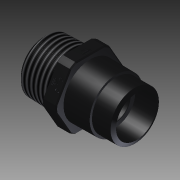
# Autodesk Inventor part: HSK-K 1.209.1201.70-Gland
Saved by Autodesk Inventor 2011 SP1 (Build 150282100, 282)
## iProperties
Created: 2018-02-18
Part Number: HSK-K 1.209.1201.70-Gland
Catalog Web Link: www.cadenas.de
Description: HSK-K NPT-Gland-Industrial cable glands
Vendor: SEALCON
Document SubType Name: Modeling
Designer: psAdmin
Manufacturer: SEALCON
Mass: 7.12094 g
Surface Area: 44.4321 cm^2
Volume: 7.12094 cm^3
Density: 1 g/cm^3
Category: PARTsolutions
Company: SEALCON
Title: HSK-K 1.209.1201.70-Gland
Author: Cadenas PARTsolutions
Comments: Industrial cable glands
PSOL_IDENT_0: {$CADENAS_DATA\23d-libs\sealcon\kabelverschraubungen\industriekabelverschraubungen\hsk_standard_kabe
PSOL_IDENT_1: lver\hsk_k\npt\hsk_k_npt_gland.prj},215 {VTYP=3D},{NB=HSK-K 1.209.1201.70-Gland},{LINA=HSK-K 1.209.1
PSOL_IDENT_2: 201.70-Gland},{NN=HSK-K NPT-Gland},{DATE=25.01.2018 07:57:44},{GEOMDATE=25.01.2018 07:44:49},{VERSIO
PSOL_IDENT_3: N=v121206082159},{LINEID=200},{LINESUBID=-1},{WBVAR=}  {NB=HSK-K 1.209.1201.70_gland},{LINA=HSK-K 1.
PSOL_IDENT_4: 209.1201.70_gland},{KT=DUMMY},{AG=1/2\" NPT},{FR=black},{GL=13},{H=27},{SW=24},{BN=1.209.1201.70},{C
PSOL_IDENT_5: OLX=0.04,0.04,0.04,0.00},{VER=2}
NN: HSK-K NPT-Gland
NT: Industrial cable glands
NB: HSK-K 1.209.1201.70-Gland
NBSYN: HSK-K $BN.-Gland
LINA: HSK-K 1.209.1201.70-Gland
AG: 1/2" NPT
FR: black
GL: 13
H: 27
SW: 24
BN: 1.209.1201.70
VER: 2
SUPPLIER: SEALCON
ARTICLENO: HSK-K 1.209.1201.70-Gland
BOMINFO: HSK-K 1.209.1201.70-Gland
CREATOR: CADENAS GmbH
Autodesk Inventor part; units mm, degrees
ref_plane "YZ Plane" through (0, 0, 0) normal (1, 0, 0) x (0, 1, 0)
ref_plane "XZ Plane" through (0, 0, 0) normal (0, 1, 0) x (-1, 0, 0)
ref_plane "XY Plane" through (0, 0, 0) normal (0, 0, 1) x (1, 0, 0)
sketch "Sketch_1" plane through (0, 0, 0) normal (0, 0, 1) x (1, 0, 0)
  line L0 (18, 0) -> (0, 0)
  line L1 (0, 0) -> (0, 8.75)
  line L2 (0, 8.75) -> (1.3401, 10.0901)
  line L3 (1.3401, 10.0901) -> (13, 10.4541)
  line L4 (13, 10.4541) -> (13, 13.2)
  line L5 (13, 13.2) -> (17.6, 13.2)
  line L6 (17.6, 13.2) -> (18, 12.8)
  line L7 (18, 12.8) -> (18, 0)
  line L8 (18, 0) -> (0, 0)
  constraints: 18 end point
revolve "Revolution1" add sketch "Sketch_1" angle 360 about axis through (18, 0, 0) along (1, 0, 0)
thread "Thread1" size "1/2" designation "1/2 - 14 NPT" standard "NPT" full length
sketch "Sketch_2" plane through (18, 0, 0) normal (1, 0, 0) x (0, 0, -1)
  line L0 (-24, -24) -> (24, -24)
  line L1 (24, -24) -> (24, 24)
  line L2 (24, 24) -> (-24, 24)
  line L3 (-24, 24) -> (-24, -24)
  line L4 (-12, -6.9282) -> (0, -13.8564)
  line L5 (0, -13.8564) -> (12, -6.9282)
  line L6 (12, -6.9282) -> (12, 6.9282)
  line L7 (12, 6.9282) -> (0, 13.8564)
  line L8 (0, 13.8564) -> (-12, 6.9282)
  line L9 (-12, 6.9282) -> (-12, -6.9282)
  constraints: 20 end point
extrude "Extrusion1" cut sketch "Sketch_2" against normal blind 5
sketch "Sketch_3" plane through (0, 0, 0) normal (0, 0, 1) x (1, 0, 0)
  line L0 (27.5, 0) -> (18, 0)
  line L1 (18, 0) -> (18, 10.325)
  line L2 (18, 10.325) -> (28, 10.225)
  line L3 (28, 10.225) -> (28, 9.35)
  line L4 (28, 9.35) -> (28.7, 9.35)
  line L5 (28.7, 9.35) -> (28.7, 7.85)
  line L6 (28.7, 7.85) -> (27.5, 7.85)
  line L7 (27.5, 7.85) -> (27.5, 0)
  line L8 (27.5, 0) -> (18, 0)
  constraints: 18 end point
revolve "Revolution2" add sketch "Sketch_3" angle 360 about axis through (27.5, 0, 0) along (1, 0, 0)
sketch "Sketch_5" plane through (0, 0, 0) normal (0, 0, 1) x (1, 0, 0)
  line L0 (28.5, 0) -> (-1, 0)
  line L1 (-1, 0) -> (-1, 7.4828)
  line L2 (-1, 7.4828) -> (0, 7.4828)
  arc A0 (0, 7.4828) -> (0.9826, 6.4829) centre (1, 7.4828) ccw
  line L3 (0.9826, 6.4829) -> (23, 6.1)
  line L4 (23, 6.1) -> (27.3, 6.1)
  arc A1 (27.3, 6.1) -> (27.5, 6.3) centre (27.3, 6.3) ccw
  line L5 (27.5, 6.3) -> (28.5, 6.3)
  line L6 (28.5, 6.3) -> (28.5, 0)
  line L7 (28.5, 0) -> (-1, 0)
  constraints: 16 end point, 4 point on circle, 2 centre point
revolve "Revolution3" cut sketch "Sketch_5" angle 360 about axis through (28.5, 0, 0) along (1, 0, 0)
sketch "Sketch_4" plane through (0, 0, 12) normal (0, 0, 1) x (1, 0, 0)
  line L0 (15.8137, 0.9977) -> (16.0537, 0.9977)
  line L1 (16.0537, 0.9977) -> (16.0537, -1.1725)
  arc A0 (16.0537, -1.1725) -> (17, -1.1725) centre (16.5269, -1.1725) ccw
  line L2 (17, -1.1725) -> (17, -1.0594)
  line L3 (17, -1.0594) -> (17.24, -1.0594)
  line L4 (17.24, -1.0594) -> (17.24, -0.936)
  line L5 (17.24, -0.936) -> (17, -0.936)
  line L6 (17, -0.936) -> (17, 1.1725)
  arc A1 (17, 1.1725) -> (16.0537, 1.1725) centre (16.5269, 1.1725) ccw
  line L7 (16.0537, 1.1725) -> (16.0537, 1.1211)
  line L8 (16.0537, 1.1211) -> (15.8137, 1.1211)
  line L9 (15.8137, 1.1211) -> (15.8137, 0.9977)
  arc A2 (16.1772, -1.1725) -> (16.8766, -1.1725) centre (16.5269, -1.1725) ccw
  line L10 (16.8766, -1.1725) -> (16.8766, -1.0594)
  line L11 (16.8766, -1.0594) -> (16.3596, -1.0594)
  line L12 (16.3596, -1.0594) -> (16.3596, -1.1211)
  line L13 (16.3596, -1.1211) -> (16.2937, -1.1211)
  line L14 (16.2937, -1.1211) -> (16.2937, -0.936)
  line L15 (16.2937, -0.936) -> (16.8766, -0.936)
  line L16 (16.8766, -0.936) -> (16.8766, 1.1725)
  arc A3 (16.8766, 1.1725) -> (16.1772, 1.1725) centre (16.5269, 1.1725) ccw
  line L17 (16.1772, 1.1725) -> (16.1772, 1.1211)
  line L18 (16.1772, 1.1211) -> (16.76, 1.1211)
  line L19 (16.76, 1.1211) -> (16.76, 0.9977)
  line L20 (16.76, 0.9977) -> (16.5598, 0.9977)
  line L21 (16.5598, 0.9977) -> (16.5598, 0.936)
  line L22 (16.5598, 0.936) -> (16.76, 0.936)
  line L23 (16.76, 0.936) -> (16.76, 0.8194)
  line L24 (16.76, 0.8194) -> (16.2937, 0.8194)
  line L25 (16.2937, 0.8194) -> (16.2937, 0.936)
  line L26 (16.2937, 0.936) -> (16.494, 0.936)
  line L27 (16.494, 0.936) -> (16.494, 0.9977)
  line L28 (16.494, 0.9977) -> (16.1772, 0.9977)
  line L29 (16.1772, 0.9977) -> (16.1772, -1.1725)
  constraints: 60 end point, 8 point on circle, 4 centre point
extrude "Extrusion2" cut sketch "Sketch_4" against normal blind 0.2
sketch "Sketch_8" plane through (0, 0, 12) normal (0, 0, 1) x (1, 0, 0)
  line L0 (16.2937, -0.8743) -> (16.3596, -0.8743)
  line L1 (16.3596, -0.8743) -> (16.3596, -0.8125)
  line L2 (16.3596, -0.8125) -> (16.494, -0.8125)
  line L3 (16.494, -0.8125) -> (16.494, -0.8743)
  line L4 (16.494, -0.8743) -> (16.5598, -0.8743)
  line L5 (16.5598, -0.8743) -> (16.5598, -0.8125)
  line L6 (16.5598, -0.8125) -> (16.6942, -0.8125)
  line L7 (16.6942, -0.8125) -> (16.6942, -0.8743)
  line L8 (16.6942, -0.8743) -> (16.76, -0.8743)
  line L9 (16.76, -0.8743) -> (16.76, -0.696)
  line L10 (16.76, -0.696) -> (16.2937, -0.696)
  line L11 (16.2937, -0.696) -> (16.2937, -0.8743)
  constraints: 24 end point
extrude "Extrusion3" cut sketch "Sketch_8" against normal blind 0.2
sketch "Sketch_9" plane through (0, 0, 12) normal (0, 0, 1) x (1, 0, 0)
  line L0 (16.2937, -0.264) -> (16.6942, -0.264)
  line L1 (16.6942, -0.264) -> (16.6942, -0.3257)
  line L2 (16.6942, -0.3257) -> (16.2937, -0.3257)
  line L3 (16.2937, -0.3257) -> (16.2937, -0.4491)
  line L4 (16.2937, -0.4491) -> (16.6942, -0.4491)
  line L5 (16.6942, -0.4491) -> (16.6942, -0.5108)
  line L6 (16.6942, -0.5108) -> (16.2937, -0.5108)
  line L7 (16.2937, -0.5108) -> (16.2937, -0.6343)
  line L8 (16.2937, -0.6343) -> (16.76, -0.6343)
  line L9 (16.76, -0.6343) -> (16.76, -0.1474)
  line L10 (16.76, -0.1474) -> (16.2937, -0.1474)
  line L11 (16.2937, -0.1474) -> (16.2937, -0.264)
  constraints: 24 end point
extrude "Extrusion4" cut sketch "Sketch_9" against normal blind 0.2
sketch "Sketch_10" plane through (0, 0, 12) normal (0, 0, 1) x (1, 0, 0)
  line L0 (16.2937, 0.0377) -> (16.2937, -0.0857)
  line L1 (16.2937, -0.0857) -> (16.76, -0.0857)
  line L2 (16.76, -0.0857) -> (16.76, 0.4011)
  line L3 (16.76, 0.4011) -> (16.2937, 0.4011)
  line L4 (16.2937, 0.4011) -> (16.2937, 0.2846)
  line L5 (16.2937, 0.2846) -> (16.6942, 0.2846)
  line L6 (16.6942, 0.2846) -> (16.6942, 0.2229)
  line L7 (16.6942, 0.2229) -> (16.2937, 0.2229)
  line L8 (16.2937, 0.2229) -> (16.2937, 0.0994)
  line L9 (16.2937, 0.0994) -> (16.6942, 0.0994)
  line L10 (16.6942, 0.0994) -> (16.6942, 0.0377)
  line L11 (16.6942, 0.0377) -> (16.2937, 0.0377)
  constraints: 24 end point
extrude "Extrusion5" cut sketch "Sketch_10" against normal blind 0.2
sketch "Sketch_11" plane through (0, 0, 12) normal (0, 0, 1) x (1, 0, 0)
  line L0 (16.2937, 0.7577) -> (16.2937, 0.4628)
  line L1 (16.2937, 0.4628) -> (16.76, 0.4628)
  line L2 (16.76, 0.4628) -> (16.76, 0.5794)
  line L3 (16.76, 0.5794) -> (16.3596, 0.5794)
  line L4 (16.3596, 0.5794) -> (16.3596, 0.6411)
  line L5 (16.3596, 0.6411) -> (16.76, 0.6411)
  line L6 (16.76, 0.6411) -> (16.76, 0.7577)
  line L7 (16.76, 0.7577) -> (16.2937, 0.7577)
  constraints: 16 end point
extrude "Extrusion6" cut sketch "Sketch_11" against normal blind 0.2
sketch "Sketch_12" plane through (0, -10.3923, 6) normal (0, 0.8660254, -0.5) x (1, 0, 0)
  arc A0 (16.2286, -1.6686) -> (16.2286, -2.0114) centre (16.2286, -1.84) ccw
  line L0 (16.2286, -2.0114) -> (16.7429, -2.0114)
  line L1 (16.7429, -2.0114) -> (16.7429, -1.9428)
  line L2 (16.7429, -1.9428) -> (16.2286, -1.9428)
  arc A1 (16.2286, -1.7371) -> (16.2286, -1.9428) centre (16.2286, -1.84) ccw
  line L3 (16.2286, -1.7371) -> (16.7429, -1.7371)
  line L4 (16.7429, -1.7371) -> (16.7429, -1.6686)
  line L5 (16.7429, -1.6686) -> (16.2286, -1.6686)
  constraints: 12 end point, 4 point on circle, 2 centre point
extrude "Extrusion7" cut sketch "Sketch_12" along normal blind 0.2
sketch "Sketch_13" plane through (0, -10.3923, 6) normal (0, 0.8660254, -0.5) x (1, 0, 0)
  line L0 (15.8892, 1.8857) -> (15.8892, 1.7829)
  line L1 (15.8892, 1.7829) -> (16.7086, 1.7829)
  arc A0 (16.7086, 1.7829) -> (16.7732, 1.8743) centre (16.7086, 1.8514) ccw
  arc A1 (16.7732, 1.8743) -> (16.3692, 2.16) centre (16.3692, 1.7314) ccw
  arc A2 (16.3692, 2.16) -> (16.093, 2.0591) centre (16.3692, 1.7314) ccw
  line L2 (16.093, 2.0591) -> (16.166, 1.986)
  arc A3 (16.3149, 2.0526) -> (16.166, 1.986) centre (16.3692, 1.7314) ccw
  arc A4 (16.3349, 2.0357) -> (16.3149, 2.0526) centre (16.3178, 2.0357) ccw
  line L3 (16.3349, 2.0357) -> (16.3349, 1.9029)
  arc A5 (16.3178, 1.8857) -> (16.3349, 1.9029) centre (16.3178, 1.9029) ccw
  line L4 (16.3178, 1.8857) -> (15.8892, 1.8857)
  arc A6 (16.4378, 1.9029) -> (16.4549, 1.8857) centre (16.4549, 1.9029) ccw
  line L5 (16.4549, 1.8857) -> (16.6257, 1.8857)
  arc A7 (16.6257, 1.8857) -> (16.64, 1.9124) centre (16.6257, 1.9029) ccw
  arc A8 (16.64, 1.9124) -> (16.4597, 2.0443) centre (16.3692, 1.7314) ccw
  arc A9 (16.4597, 2.0443) -> (16.4378, 2.0279) centre (16.4549, 2.0279) ccw
  line L6 (16.4378, 2.0279) -> (16.4378, 1.9029)
  constraints: 20 point on circle, 14 end point, 10 centre point
extrude "Extrusion8" cut sketch "Sketch_13" along normal blind 0.2
sketch "Sketch_28" plane through (0, -10.3923, 6) normal (0, 0.8660254, -0.5) x (1, 0, 0)
  line L0 (15.7829, -1.1886) -> (15.7829, -1.5314)
  line L1 (15.7829, -1.5314) -> (16.4686, -1.5314)
  line L2 (16.4686, -1.5314) -> (16.4686, -1.4629)
  line L3 (16.4686, -1.4629) -> (15.8515, -1.4629)
  line L4 (15.8515, -1.4629) -> (15.8515, -1.1886)
  line L5 (15.8515, -1.1886) -> (15.7829, -1.1886)
  constraints: 12 end point
extrude "Extrusion9" cut sketch "Sketch_28" along normal blind 0.2
sketch "Sketch_29" plane through (0, -10.3923, 6) normal (0, 0.8660254, -0.5) x (1, 0, 0)
  circle A0 centre (16.2629, -1.6) radius 0.7371
  circle A1 centre (16.2629, -1.6) radius 0.7028
  constraints: 2 centre point
extrude "Extrusion10" cut sketch "Sketch_29" along normal blind 0.2
sketch "Sketch_14" plane through (0, -10.3923, 6) normal (0, 0.8660254, -0.5) x (1, 0, 0)
  arc A0 (16.0526, 1.6286) -> (15.9923, 1.5274) centre (16.0526, 1.56) ccw
  arc A1 (15.9923, 1.5274) -> (16.2442, 1.3215) centre (16.3692, 1.7314) ccw
  arc A2 (16.2442, 1.3215) -> (16.2663, 1.3379) centre (16.2492, 1.3379) ccw
  line L0 (16.2663, 1.3379) -> (16.2663, 1.4103)
  arc A3 (16.2663, 1.4103) -> (16.2552, 1.4263) centre (16.2492, 1.4103) ccw
  arc A4 (16.1439, 1.4962) -> (16.2552, 1.4263) centre (16.3692, 1.7314) ccw
  arc A5 (16.1558, 1.5257) -> (16.1439, 1.4962) centre (16.1558, 1.5086) ccw
  line L1 (16.1558, 1.5257) -> (16.2639, 1.5257)
  arc A6 (16.3124, 1.5057) -> (16.2639, 1.5257) centre (16.2639, 1.4572) ccw
  line L2 (16.3124, 1.5057) -> (16.4649, 1.3531)
  arc A7 (16.4649, 1.3531) -> (16.5409, 1.3388) centre (16.5134, 1.4016) ccw
  arc A8 (16.5409, 1.3388) -> (16.746, 1.5274) centre (16.3692, 1.7314) ccw
  arc A9 (16.746, 1.5274) -> (16.6857, 1.6286) centre (16.6857, 1.56) ccw
  line L3 (16.6857, 1.6286) -> (16.592, 1.6286)
  arc A10 (16.592, 1.6286) -> (16.5749, 1.6115) centre (16.592, 1.6115) ccw
  line L4 (16.5749, 1.6115) -> (16.5749, 1.5429)
  arc A11 (16.5749, 1.5429) -> (16.592, 1.5257) centre (16.592, 1.5429) ccw
  line L5 (16.592, 1.5257) -> (16.6217, 1.5257)
  arc A12 (16.5321, 1.4494) -> (16.6217, 1.5257) centre (16.3692, 1.7314) ccw
  arc A13 (16.5114, 1.4521) -> (16.5321, 1.4494) centre (16.5235, 1.4642) ccw
  line L6 (16.5114, 1.4521) -> (16.355, 1.6085)
  arc A14 (16.355, 1.6085) -> (16.3065, 1.6286) centre (16.3065, 1.56) ccw
  line L7 (16.3065, 1.6286) -> (16.0526, 1.6286)
  constraints: 30 point on circle, 16 end point, 15 centre point
extrude "Extrusion11" cut sketch "Sketch_14" along normal blind 0.2
sketch "Sketch_15" plane through (0, -10.3923, 6) normal (0, 0.8660254, -0.5) x (1, 0, 0)
  arc A0 (15.8864, 2.2656) -> (16.8519, 2.2656) centre (16.3692, 1.7314) ccw
  line L0 (16.8519, 2.2656) -> (16.7426, 2.1563)
  arc A1 (15.9957, 2.1563) -> (16.7426, 2.1563) centre (16.3692, 1.7314) ccw
  line L1 (15.9957, 2.1563) -> (15.8864, 2.2656)
  constraints: 4 end point, 4 point on circle, 2 centre point
extrude "Extrusion12" cut sketch "Sketch_15" along normal blind 0.2
sketch "Sketch_16" plane through (0, 0, 12) normal (0, 0, 1) x (1, 0, 0)
  arc A0 (15, 0.914) -> (15.025, 0.889) centre (15.025, 0.914) ccw
  line L0 (15.025, 0.889) -> (15.181, 0.889)
  line L1 (15.181, 0.889) -> (15.181, 0.7925)
  arc A1 (15.181, 0.7925) -> (15.2875, 0.686) centre (15.2875, 0.7925) ccw
  line L2 (15.2875, 0.686) -> (15.3715, 0.686)
  arc A2 (15.3715, 0.686) -> (15.478, 0.7925) centre (15.3715, 0.7925) ccw
  line L3 (15.478, 0.7925) -> (15.478, 0.935)
  arc A3 (15.478, 0.935) -> (15.453, 0.96) centre (15.453, 0.935) ccw
  line L4 (15.453, 0.96) -> (15.025, 0.96)
  arc A4 (15.025, 0.96) -> (15, 0.935) centre (15.025, 0.935) ccw
  line L5 (15, 0.935) -> (15, 0.914)
  line L6 (15.252, 0.889) -> (15.252, 0.8103)
  arc A5 (15.252, 0.8103) -> (15.3052, 0.757) centre (15.3053, 0.8103) ccw
  line L7 (15.3052, 0.757) -> (15.3538, 0.757)
  arc A6 (15.3538, 0.757) -> (15.407, 0.8103) centre (15.3537, 0.8103) ccw
  line L8 (15.407, 0.8103) -> (15.407, 0.889)
  line L9 (15.407, 0.889) -> (15.252, 0.889)
  constraints: 20 end point, 14 point on circle, 7 centre point
extrude "Extrusion13" cut sketch "Sketch_16" against normal blind 0.2
sketch "Sketch_17" plane through (0, 0, 12) normal (0, 0, 1) x (1, 0, 0)
  arc A0 (15.0011, 0.3808) -> (15.037, 0.345) centre (15.037, 0.3808) ccw
  line L0 (15.037, 0.345) -> (15.2754, 0.345)
  arc A1 (15.2754, 0.345) -> (15.3561, 0.4257) centre (15.2754, 0.4257) ccw
  line L1 (15.3561, 0.4257) -> (15.3561, 0.5664)
  arc A2 (15.3561, 0.5664) -> (15.2843, 0.5664) centre (15.3202, 0.5664) ccw
  line L2 (15.2843, 0.5664) -> (15.2843, 0.4257)
  arc A3 (15.2754, 0.4167) -> (15.2843, 0.4257) centre (15.2754, 0.4257) ccw
  line L3 (15.2754, 0.4167) -> (15.2346, 0.4167)
  line L4 (15.2346, 0.4167) -> (15.2346, 0.5381)
  arc A4 (15.2346, 0.5381) -> (15.1539, 0.6188) centre (15.1539, 0.5381) ccw
  line L5 (15.1539, 0.6188) -> (15.0818, 0.6188)
  arc A5 (15.0818, 0.6188) -> (15.0011, 0.5381) centre (15.0818, 0.5381) ccw
  line L6 (15.0011, 0.5381) -> (15.0011, 0.3808)
  line L7 (15.0728, 0.4167) -> (15.1629, 0.4167)
  line L8 (15.1629, 0.4167) -> (15.1629, 0.5381)
  arc A6 (15.1629, 0.5381) -> (15.1539, 0.5471) centre (15.1539, 0.5381) ccw
  line L9 (15.1539, 0.5471) -> (15.0818, 0.5471)
  arc A7 (15.0818, 0.5471) -> (15.0728, 0.5381) centre (15.0818, 0.5381) ccw
  line L10 (15.0728, 0.5381) -> (15.0728, 0.4167)
  constraints: 22 end point, 16 point on circle, 8 centre point
extrude "Extrusion14" cut sketch "Sketch_17" against normal blind 0.2
sketch "Sketch_18" plane through (0, 0, 12) normal (0, 0, 1) x (1, 0, 0)
  arc A0 (15.0353, 0.2372) -> (15.0353, 0.1654) centre (15.0353, 0.2013) ccw
  line L0 (15.0353, 0.1654) -> (15.2843, 0.1654)
  line L1 (15.2843, 0.1654) -> (15.2843, 0.1204)
  arc A1 (15.2843, 0.1204) -> (15.3561, 0.1204) centre (15.3202, 0.1204) ccw
  line L2 (15.3561, 0.1204) -> (15.3561, 0.1654)
  line L3 (15.3561, 0.1654) -> (15.44, 0.1654)
  arc A2 (15.44, 0.1654) -> (15.44, 0.2372) centre (15.44, 0.2013) ccw
  line L4 (15.44, 0.2372) -> (15.3561, 0.2372)
  arc A3 (15.3561, 0.2372) -> (15.2843, 0.2372) centre (15.3202, 0.2401) ccw
  line L5 (15.2843, 0.2372) -> (15.0353, 0.2372)
  constraints: 12 end point, 8 point on circle, 4 centre point
extrude "Extrusion15" cut sketch "Sketch_18" against normal blind 0.2
sketch "Sketch_19" plane through (0, 0, 12) normal (0, 0, 1) x (1, 0, 0)
  arc A0 (15.0013, -0.212) -> (15.0263, -0.237) centre (15.0263, -0.212) ccw
  line L0 (15.0263, -0.237) -> (15.0489, -0.237)
  arc A1 (15.0489, -0.237) -> (15.0739, -0.212) centre (15.0489, -0.212) ccw
  line L1 (15.0739, -0.212) -> (15.0739, -0.0709)
  arc A2 (15.1102, -0.0346) -> (15.0739, -0.0709) centre (15.1102, -0.0709) ccw
  line L2 (15.1102, -0.0346) -> (15.1439, -0.0346)
  line L3 (15.1439, -0.0346) -> (15.1439, -0.2007)
  arc A3 (15.1439, -0.2007) -> (15.1802, -0.237) centre (15.1802, -0.2007) ccw
  line L4 (15.1802, -0.237) -> (15.2165, -0.237)
  arc A4 (15.2165, -0.237) -> (15.2165, 0.038) centre (15.2165, -0.0995) ccw
  line L5 (15.2165, 0.038) -> (15.1263, 0.038)
  arc A5 (15.1263, 0.038) -> (15.0013, -0.087) centre (15.1263, -0.087) ccw
  line L6 (15.0013, -0.087) -> (15.0013, -0.212)
  arc A6 (15.2165, -0.1644) -> (15.2165, -0.0346) centre (15.2077, -0.0995) ccw
  line L7 (15.2165, -0.0346) -> (15.2165, -0.1644)
  constraints: 16 end point, 14 point on circle, 7 centre point
extrude "Extrusion16" cut sketch "Sketch_19" against normal blind 0.2
sketch "Sketch_20" plane through (0, 0, 12) normal (0, 0, 1) x (1, 0, 0)
  arc A0 (15.037, -0.3091) -> (15.037, -0.3809) centre (15.037, -0.345) ccw
  line L0 (15.037, -0.3809) -> (15.2843, -0.3809)
  line L1 (15.2843, -0.3809) -> (15.2843, -0.4664)
  arc A1 (15.2395, -0.5113) -> (15.2843, -0.4664) centre (15.2395, -0.4664) ccw
  line L2 (15.2395, -0.5113) -> (15.037, -0.5113)
  arc A2 (15.037, -0.5113) -> (15.037, -0.583) centre (15.037, -0.5471) ccw
  line L3 (15.037, -0.583) -> (15.2395, -0.583)
  arc A3 (15.2395, -0.583) -> (15.3561, -0.4664) centre (15.2395, -0.4664) ccw
  line L4 (15.3561, -0.4664) -> (15.3561, -0.345)
  arc A4 (15.3561, -0.345) -> (15.3202, -0.3091) centre (15.3202, -0.345) ccw
  line L5 (15.3202, -0.3091) -> (15.037, -0.3091)
  constraints: 12 end point, 10 point on circle, 5 centre point
extrude "Extrusion17" cut sketch "Sketch_20" against normal blind 0.2
sketch "Sketch_21" plane through (0, 0, 12) normal (0, 0, 1) x (1, 0, 0)
  arc A0 (15.0353, -0.6946) -> (15.0353, -0.7664) centre (15.0353, -0.7305) ccw
  line L0 (15.0353, -0.7664) -> (15.2843, -0.7664)
  line L1 (15.2843, -0.7664) -> (15.2843, -0.8114)
  arc A1 (15.2843, -0.8114) -> (15.3561, -0.8114) centre (15.3202, -0.8114) ccw
  line L2 (15.3561, -0.8114) -> (15.3561, -0.7664)
  line L3 (15.3561, -0.7664) -> (15.44, -0.7664)
  arc A2 (15.44, -0.7664) -> (15.44, -0.6946) centre (15.44, -0.7305) ccw
  line L4 (15.44, -0.6946) -> (15.3561, -0.6946)
  arc A3 (15.3561, -0.6946) -> (15.2843, -0.6946) centre (15.3202, -0.6946) ccw
  line L5 (15.2843, -0.6946) -> (15.0353, -0.6946)
  constraints: 12 end point, 8 point on circle, 4 centre point
extrude "Extrusion18" cut sketch "Sketch_21" against normal blind 0.2
sketch "Sketch_22" plane through (0, -10.3923, 6) normal (0, 0.8660254, -0.5) x (1, 0, 0)
  line L0 (14.8285, 0.0411) -> (14.8285, -0.0411)
  line L1 (14.8285, -0.0411) -> (15.3428, -0.2571)
  line L2 (15.3428, -0.2571) -> (15.3428, -0.1679)
  line L3 (15.3428, -0.1679) -> (14.9431, 0)
  line L4 (14.9431, 0) -> (15.3428, 0.1679)
  line L5 (15.3428, 0.1679) -> (15.3428, 0.2571)
  line L6 (15.3428, 0.2571) -> (14.8285, 0.0411)
  constraints: 14 end point
extrude "Extrusion19" cut sketch "Sketch_22" along normal blind 0.2
sketch "Sketch_23" plane through (0, -10.3923, 6) normal (0, 0.8660254, -0.5) x (1, 0, 0)
  line L0 (14.4583, -0.5554) -> (14.9725, -0.5554)
  line L1 (14.9725, -0.5554) -> (14.9725, -0.3394)
  arc A0 (14.9725, -0.3394) -> (14.8183, -0.1851) centre (14.8183, -0.3394) ccw
  line L2 (14.8183, -0.1851) -> (14.6125, -0.1851)
  arc A1 (14.6125, -0.1851) -> (14.4583, -0.3394) centre (14.6125, -0.3394) ccw
  line L3 (14.4583, -0.3394) -> (14.4583, -0.5554)
  line L4 (14.5406, -0.3394) -> (14.5406, -0.4731)
  line L5 (14.5406, -0.4731) -> (14.8903, -0.4731)
  line L6 (14.8903, -0.4731) -> (14.8903, -0.3394)
  arc A2 (14.8903, -0.3394) -> (14.8183, -0.2674) centre (14.8183, -0.3394) ccw
  line L7 (14.8183, -0.2674) -> (14.6125, -0.2674)
  arc A3 (14.6125, -0.2674) -> (14.5406, -0.3394) centre (14.6125, -0.3394) ccw
  constraints: 16 end point, 8 point on circle, 4 centre point
extrude "Extrusion20" cut sketch "Sketch_23" along normal blind 0.2
sketch "Sketch_24" plane through (0, -10.3923, 6) normal (0, 0.8660254, -0.5) x (1, 0, 0)
  line L0 (14.4583, 0.5554) -> (14.4583, 0.1851)
  line L1 (14.4583, 0.1851) -> (14.9725, 0.1851)
  line L2 (14.9725, 0.1851) -> (14.9725, 0.5554)
  line L3 (14.9725, 0.5554) -> (14.8903, 0.5554)
  line L4 (14.8903, 0.5554) -> (14.8903, 0.2674)
  line L5 (14.8903, 0.2674) -> (14.7565, 0.2674)
  line L6 (14.7565, 0.2674) -> (14.7565, 0.4628)
  line L7 (14.7565, 0.4628) -> (14.6743, 0.4628)
  line L8 (14.6743, 0.4628) -> (14.6743, 0.2674)
  line L9 (14.6743, 0.2674) -> (14.5406, 0.2674)
  line L10 (14.5406, 0.2674) -> (14.5406, 0.5554)
  line L11 (14.5406, 0.5554) -> (14.4583, 0.5554)
  constraints: 24 end point
extrude "Extrusion21" cut sketch "Sketch_24" along normal blind 0.2
sketch "Sketch_25" plane through (0, -10.3923, 6) normal (0, 0.8660254, -0.5) x (1, 0, 0)
  line L0 (13.8, -1.0285) -> (14.2131, -1.0285)
  arc A0 (14.2131, -1.0285) -> (14.6205, -1.186) centre (14.4583, -1) ccw
  line L1 (14.6205, -1.186) -> (15.785, -0.1705)
  arc A1 (15.785, -0.1705) -> (15.785, 0.1705) centre (15.6362, 0) ccw
  line L2 (15.785, 0.1705) -> (14.6205, 1.186)
  arc A2 (14.6205, 1.186) -> (14.2131, 1.0285) centre (14.4583, 1) ccw
  line L3 (14.2131, 1.0285) -> (13.8, 1.0285)
  line L4 (13.8, 1.0285) -> (13.8, -1.0285)
  line L5 (14.2937, 1) -> (14.2937, -1)
  arc A3 (14.2937, -1) -> (14.5664, -1.124) centre (14.4583, -1) ccw
  line L6 (14.5664, -1.124) -> (15.7309, -0.1085)
  arc A4 (15.7309, -0.1085) -> (15.7309, 0.1085) centre (15.6362, 0) ccw
  line L7 (15.7309, 0.1085) -> (14.5664, 1.124)
  arc A5 (14.5664, 1.124) -> (14.2937, 1) centre (14.4583, 1) ccw
  line L8 (13.8823, -0.9463) -> (14.2114, -0.9463)
  line L9 (14.2114, -0.9463) -> (14.2114, 0.9463)
  line L10 (14.2114, 0.9463) -> (13.8823, 0.9463)
  line L11 (13.8823, 0.9463) -> (13.8823, -0.9463)
  constraints: 24 end point, 12 point on circle, 6 centre point
extrude "Extrusion22" cut sketch "Sketch_25" along normal blind 0.2
sketch "Sketch_26" plane through (0, 0, 0) normal (0, 0, 1) x (1, 0, 0)
  line L0 (36, 0) -> (28.7, 0)
  line L1 (28.7, 9.35) -> (28.7, 7.85)
  line L2 (28.7, 7.85) -> (35.7553, 7.85)
  line L3 (35.7553, 7.85) -> (35.1586, 9.2557)
  arc A0 (35.1586, 9.2557) -> (35.1126, 9.35) centre (34.2381, 8.865) ccw
  line L4 (35.1126, 9.35) -> (28.7, 9.35)
  constraints: 10 end point, 2 point on circle, 1 centre point
revolve "Revolution4" add sketch "Sketch_26" angle 360 about axis through (36, 0, 0) along (1, 0, 0)
sketch "Sketch_27" plane through (0, 10.3923, -6) normal (0, 0.8660254, -0.5) x (1, 0, 0)
  arc A0 (14.9269, 2.0546) -> (14.9269, 1.9501) centre (14.9269, 2.0023) ccw
  line L0 (14.9269, 1.9501) -> (15.6916, 1.9501)
  arc A1 (15.6916, 1.9501) -> (15.7316, 1.9901) centre (15.6916, 1.9901) ccw
  arc A2 (15.7316, 1.9901) -> (15.7124, 2.028) centre (15.6905, 1.9931) ccw
  arc A3 (15.5286, 2.2418) -> (15.7124, 2.028) centre (16.0258, 2.4833) ccw
  arc A4 (15.5286, 2.2418) -> (15.4441, 2.2446) centre (15.4853, 2.2096) ccw
  arc A5 (15.4441, 2.2446) -> (15.4424, 2.2057) centre (15.479, 2.2236) ccw
  arc A6 (15.4424, 2.2057) -> (15.5429, 2.0546) centre (16.0503, 2.5011) ccw
  line L1 (15.5429, 2.0546) -> (14.9269, 2.0546)
  constraints: 14 point on circle, 7 centre point, 4 end point
extrude "Extrusion23" cut sketch "Sketch_27" against normal blind 0.2
sketch "Sketch_30" plane through (0, 10.3923, -6) normal (0, 0.8660254, -0.5) x (1, 0, 0)
  line L0 (14.8375, 1.6917) -> (15.6169, 1.2417)
  line L1 (15.6169, 1.2417) -> (15.6794, 1.35)
  line L2 (15.6794, 1.35) -> (14.9, 1.8)
  line L3 (14.9, 1.8) -> (14.8375, 1.6917)
  constraints: 8 end point
extrude "Extrusion24" cut sketch "Sketch_30" against normal blind 0.2
sketch "Sketch_31" plane through (0, 10.3923, -6) normal (0, 0.8660254, -0.5) x (1, 0, 0)
  line L0 (14.8769, 1.2243) -> (14.8769, 0.7117)
  arc A0 (14.8769, 0.7117) -> (14.9272, 0.6617) centre (14.9269, 0.7117) ccw
  arc A1 (14.9272, 0.6617) -> (14.9774, 0.7117) centre (14.9274, 0.7117) ccw
  line L1 (14.9774, 0.7117) -> (14.9774, 1.0792)
  line L2 (14.9774, 1.0792) -> (14.9965, 1.0664)
  line L3 (14.9965, 1.0664) -> (15.0172, 1.0502)
  line L4 (15.0172, 1.0502) -> (15.0405, 1.0287)
  line L5 (15.0405, 1.0287) -> (15.0649, 1.0026)
  line L6 (15.0649, 1.0026) -> (15.0905, 0.9737)
  line L7 (15.0905, 0.9737) -> (15.1855, 0.8627)
  line L8 (15.1855, 0.8627) -> (15.221, 0.8232)
  line L9 (15.221, 0.8232) -> (15.2628, 0.7798)
  line L10 (15.2628, 0.7798) -> (15.3059, 0.7403)
  line L11 (15.3059, 0.7403) -> (15.3324, 0.7197)
  line L12 (15.3324, 0.7197) -> (15.3549, 0.7047)
  line L13 (15.3549, 0.7047) -> (15.3898, 0.686)
  line L14 (15.3898, 0.686) -> (15.4255, 0.6729)
  line L15 (15.4255, 0.6729) -> (15.4596, 0.6654)
  line L16 (15.4596, 0.6654) -> (15.5135, 0.6635)
  line L17 (15.5135, 0.6635) -> (15.5683, 0.6736)
  line L18 (15.5683, 0.6736) -> (15.6093, 0.6914)
  line L19 (15.6093, 0.6914) -> (15.6402, 0.7125)
  line L20 (15.6402, 0.7125) -> (15.6753, 0.7475)
  line L21 (15.6753, 0.7475) -> (15.6967, 0.7788)
  line L22 (15.6967, 0.7788) -> (15.715, 0.8194)
  line L23 (15.715, 0.8194) -> (15.7225, 0.8454)
  line L24 (15.7225, 0.8454) -> (15.7288, 0.8806)
  line L25 (15.7288, 0.8806) -> (15.7316, 0.9224)
  line L26 (15.7316, 0.9224) -> (15.7302, 0.9633)
  line L27 (15.7302, 0.9633) -> (15.7218, 1.0163)
  line L28 (15.7218, 1.0163) -> (15.7064, 1.0619)
  line L29 (15.7064, 1.0619) -> (15.6788, 1.1091)
  line L30 (15.6788, 1.1091) -> (15.6399, 1.1487)
  line L31 (15.6399, 1.1487) -> (15.6097, 1.1689)
  line L32 (15.6097, 1.1689) -> (15.5807, 1.1828)
  line L33 (15.5807, 1.1828) -> (15.5502, 1.1931)
  arc A2 (15.5502, 1.1931) -> (15.5194, 1.0928) centre (15.5316, 1.1439) ccw
  line L34 (15.5194, 1.0928) -> (15.5388, 1.0878)
  line L35 (15.5388, 1.0878) -> (15.5533, 1.0823)
  line L36 (15.5533, 1.0823) -> (15.5844, 1.0645)
  line L37 (15.5844, 1.0645) -> (15.6077, 1.0428)
  line L38 (15.6077, 1.0428) -> (15.6258, 1.0163)
  line L39 (15.6258, 1.0163) -> (15.6392, 0.9812)
  line L40 (15.6392, 0.9812) -> (15.6446, 0.9459)
  line L41 (15.6446, 0.9459) -> (15.6352, 0.868)
  line L42 (15.6352, 0.868) -> (15.6057, 0.8182)
  line L43 (15.6057, 0.8182) -> (15.552, 0.7802)
  line L44 (15.552, 0.7802) -> (15.4976, 0.7703)
  line L45 (15.4976, 0.7703) -> (15.4551, 0.7763)
  line L46 (15.4551, 0.7763) -> (15.4227, 0.7884)
  line L47 (15.4227, 0.7884) -> (15.3829, 0.8113)
  line L48 (15.3829, 0.8113) -> (15.3417, 0.8437)
  line L49 (15.3417, 0.8437) -> (15.2198, 0.9728)
  line L50 (15.2198, 0.9728) -> (15.1656, 1.0378)
  line L51 (15.1656, 1.0378) -> (15.1422, 1.0645)
  line L52 (15.1422, 1.0645) -> (15.0943, 1.1145)
  line L53 (15.0943, 1.1145) -> (15.058, 1.1473)
  line L54 (15.058, 1.1473) -> (15.0265, 1.1712)
  line L55 (15.0265, 1.1712) -> (14.9905, 1.1934)
  line L56 (14.9905, 1.1934) -> (14.9578, 1.2089)
  line L57 (14.9578, 1.2089) -> (14.9215, 1.2204)
  line L58 (14.9215, 1.2204) -> (14.8989, 1.2238)
  line L59 (14.8989, 1.2238) -> (14.8769, 1.2243)
  constraints: 120 end point, 6 point on circle, 3 centre point
extrude "Extrusion25" cut sketch "Sketch_31" against normal blind 0.2
sketch "Sketch_32" plane through (0, 10.3923, -6) normal (0, 0.8660254, -0.5) x (1, 0, 0)
  line L0 (15.6, 0.2) -> (15.85, 0.2)
  line L1 (15.85, 0.2) -> (15.85, 0.3)
  line L2 (15.85, 0.3) -> (15.6, 0.3)
  line L3 (15.6, 0.3) -> (15.6, 0.2)
  constraints: 8 end point
extrude "Extrusion26" cut sketch "Sketch_32" against normal blind 0.2
sketch "Sketch_33" plane through (0, 10.3923, -6) normal (0, 0.8660254, -0.5) x (1, 0, 0)
  line L0 (15.6, 0.4) -> (15.85, 0.4)
  line L1 (15.85, 0.4) -> (15.85, 0.5)
  line L2 (15.85, 0.5) -> (15.6, 0.5)
  line L3 (15.6, 0.5) -> (15.6, 0.4)
  constraints: 8 end point
extrude "Extrusion27" cut sketch "Sketch_33" against normal blind 0.2
sketch "Sketch_34" plane through (0, 10.3923, -6) normal (0, 0.8660254, -0.5) x (1, 0, 0)
  arc A0 (14.9269, 0.0126) -> (14.9269, -0.096) centre (14.9222, -0.0417) ccw
  line L0 (14.9269, -0.096) -> (15.6016, -0.096)
  line L1 (15.6016, -0.096) -> (14.9621, -0.447)
  arc A1 (14.9621, -0.447) -> (14.9621, -0.5556) centre (14.9795, -0.5013) ccw
  line L2 (14.9621, -0.5556) -> (15.7281, -0.5556)
  arc A2 (15.7281, -0.5556) -> (15.7133, -0.447) centre (15.716, -0.5019) ccw
  line L3 (15.7133, -0.447) -> (15.16, -0.447)
  line L4 (15.16, -0.447) -> (15.702, -0.1529)
  arc A3 (15.702, -0.1529) -> (15.7281, -0.109) centre (15.6781, -0.109) ccw
  line L5 (15.7281, -0.109) -> (15.7281, -0.0374)
  arc A4 (15.7281, -0.0374) -> (15.6781, 0.0126) centre (15.6781, -0.0374) ccw
  line L6 (15.6781, 0.0126) -> (14.9269, 0.0126)
  constraints: 14 end point, 10 point on circle, 5 centre point
extrude "Extrusion28" cut sketch "Sketch_34" against normal blind 0.2
sketch "Sketch_35" plane through (0, 10.3923, -6) normal (0, 0.8660254, -0.5) x (1, 0, 0)
  line L0 (14.9225, -0.7956) -> (15.31, -0.7956)
  line L1 (15.31, -0.7956) -> (15.31, -0.98)
  arc A0 (15.31, -0.98) -> (15.76, -0.98) centre (15.535, -0.9323) ccw
  line L2 (15.76, -0.98) -> (15.76, -0.7)
  line L3 (15.76, -0.7) -> (14.9225, -0.7)
  line L4 (14.9225, -0.7) -> (14.9225, -0.7956)
  line L5 (15.4056, -0.7956) -> (15.4056, -0.98)
  arc A1 (15.4056, -0.98) -> (15.6644, -0.98) centre (15.535, -0.9335) ccw
  line L6 (15.6644, -0.98) -> (15.6644, -0.7956)
  line L7 (15.6644, -0.7956) -> (15.4056, -0.7956)
  constraints: 16 end point, 4 point on circle, 2 centre point
extrude "Extrusion29" cut sketch "Sketch_35" against normal blind 0.2
sketch "Sketch_36" plane through (0, 10.3923, -6) normal (0, 0.8660254, -0.5) x (1, 0, 0)
  arc A0 (14.9798, -1.4403) -> (14.9798, -1.5598) centre (14.9798, -1.5) ccw
  line L0 (14.9798, -1.5598) -> (15.6305, -1.5598)
  line L1 (15.6305, -1.5598) -> (15.6305, -1.7403)
  arc A1 (15.6305, -1.7403) -> (15.75, -1.7403) centre (15.6902, -1.7403) ccw
  line L2 (15.75, -1.7403) -> (15.75, -1.2598)
  arc A2 (15.75, -1.2598) -> (15.6305, -1.2598) centre (15.6902, -1.2598) ccw
  line L3 (15.6305, -1.2598) -> (15.6305, -1.4403)
  line L4 (15.6305, -1.4403) -> (14.9798, -1.4403)
  constraints: 10 end point, 6 point on circle, 3 centre point
extrude "Extrusion30" cut sketch "Sketch_36" against normal blind 0.2
sketch "Sketch_37" plane through (0, 0, 0) normal (0, 1, 0) x (-1, 0, 0)
  line L0 (-17.6, -12) -> (-18, -11.6)
  line L1 (-18, -11.6) -> (-18.6, -11.6)
  line L2 (-18.6, -11.6) -> (-18.6, -12.6)
  line L3 (-18.6, -12.6) -> (-17.6, -12.6)
  line L4 (-17.6, -12.6) -> (-17.6, -12)
  constraints: 10 end point
extrude "Extrusion31" cut sketch "Sketch_37" along normal mid plane 14
sketch "Sketch_38" plane through (0, 0, 0) normal (0, 1, 0) x (-1, 0, 0)
  line L0 (-17.6, 12) -> (-17.6, 12.6)
  line L1 (-17.6, 12.6) -> (-18.6, 12.6)
  line L2 (-18.6, 12.6) -> (-18.6, 11.6)
  line L3 (-18.6, 11.6) -> (-18, 11.6)
  line L4 (-18, 11.6) -> (-17.6, 12)
  constraints: 10 end point
extrude "Extrusion32" cut sketch "Sketch_38" along normal mid plane 14
sketch "Sketch_39" plane through (0, 0, 0) normal (0, 0.5, 0.8660254) x (1, 0, 0)
  line L0 (17.6, 12) -> (18, 11.6)
  line L1 (18, 11.6) -> (18.6, 11.6)
  line L2 (18.6, 11.6) -> (18.6, 12.6)
  line L3 (18.6, 12.6) -> (17.6, 12.6)
  line L4 (17.6, 12.6) -> (17.6, 12)
  constraints: 10 end point
extrude "Extrusion33" cut sketch "Sketch_39" along normal mid plane 14
sketch "Sketch_40" plane through (0, 0, 0) normal (0, 0.5, 0.8660254) x (1, 0, 0)
  line L0 (17.6, -12) -> (17.6, -12.6)
  line L1 (17.6, -12.6) -> (18.6, -12.6)
  line L2 (18.6, -12.6) -> (18.6, -11.6)
  line L3 (18.6, -11.6) -> (18, -11.6)
  line L4 (18, -11.6) -> (17.6, -12)
  constraints: 10 end point
extrude "Extrusion34" cut sketch "Sketch_40" along normal mid plane 14
sketch "Sketch_41" plane through (0, 0, 0) normal (0, -0.5, 0.8660254) x (1, 0, 0)
  line L0 (17.6, 12) -> (18, 11.6)
  line L1 (18, 11.6) -> (18.6, 11.6)
  line L2 (18.6, 11.6) -> (18.6, 12.6)
  line L3 (18.6, 12.6) -> (17.6, 12.6)
  line L4 (17.6, 12.6) -> (17.6, 12)
  constraints: 10 end point
extrude "Extrusion35" cut sketch "Sketch_41" along normal mid plane 14
sketch "Sketch_42" plane through (0, 0, 0) normal (0, -0.5, 0.8660254) x (1, 0, 0)
  line L0 (17.6, -12) -> (17.6, -12.6)
  line L1 (17.6, -12.6) -> (18.6, -12.6)
  line L2 (18.6, -12.6) -> (18.6, -11.6)
  line L3 (18.6, -11.6) -> (18, -11.6)
  line L4 (18, -11.6) -> (17.6, -12)
  constraints: 10 end point
extrude "Extrusion36" cut sketch "Sketch_42" along normal mid plane 14
ref_plane "IP1_XY" through (0, 0, 0) normal (1, 0, 0) x (0, 0, -1)
ref_plane "IP1_YZ" through (0, 0, 0) normal (0, 0, -1) x (0, 1, 0)
ref_plane "IP1_ZX" through (0, 0, 0) normal (0, 1, 0) x (1, 0, 0)
ref_plane "IP2_XY" through (25.5, 0, 0) normal (1, 0, 0) x (0, 0, -1)
ref_plane "IP2_YZ" through (25.5, 0, 0) normal (0, 0, -1) x (0, 1, 0)
ref_plane "IP2_ZX" through (25.5, 0, 0) normal (0, 1, 0) x (1, 0, 0)
body "Solid1"
